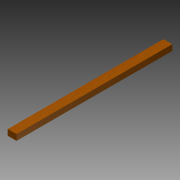
# Autodesk Inventor part: Transverse_Bottom
Saved by Autodesk Inventor 2014 SP1 (Build 180222100, 222)
## iProperties
Created: 2014-02-22
Part Number: Transverse_Bottom
Material: Wood
Document SubType Name: Modeling
Designer: tuleu
Density: 0.570257 g/cm^3
Appearance: Yellow Pine - Solid Natural Low Gloss
Author: tuleu
Autodesk Inventor part; units mm, degrees
ref_plane "YZ Plane" through (0, 0, 0) normal (1, 0, 0) x (0, 1, 0)
ref_plane "XZ Plane" through (0, 0, 0) normal (0, 1, 0) x (-1, 0, 0)
ref_plane "XY Plane" through (0, 0, 0) normal (0, 0, 1) x (1, 0, 0)
sketch "Sketch1" plane through (0, 0, 0) normal (0, 0, 1) x (1, 0, 0)
  line L0 (0, -633) -> (0, 433)
  line L1 (0, 433) -> (-60, 433)
  line L2 (-60, 433) -> (-60, -633)
  line L3 (-60, -633) -> (0, -633)
  point P0 (0, 0)
  dimension "d0" = 60
  constraints: 8 end point, 2 parallel, 1 perpendicular, 1 vertical, 3 other
  measures "d0" distance between parallel lines of L0 L2
extrude "Extrusion1" add sketch "Sketch1" along normal blind 40
body "Solid1"
